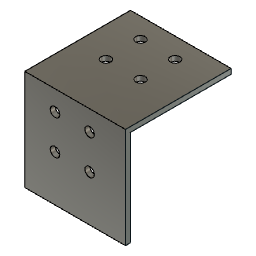
L brackets for Motors v5 (Autodesk Fusion 360 design; units mm, degrees)
Autodesk Fusion 360 part; units mm, degrees
sketch "Sketch1" plane through (0, 0, 0) normal (1, 0, 0) x (0, 1, 0)
  line L0 (0, 0) -> (2.54, 0)
  line L1 (2.54, 0) -> (2.54, 50.8)
  line L2 (2.54, 50.8) -> (0, 50.8)
  line L3 (0, 50.8) -> (0, 0)
  line L4 (0, 50.8) -> (53.34, 50.8)
  line L5 (53.34, 50.8) -> (53.34, 48.26)
  line L6 (53.34, 48.26) -> (0, 48.26)
  line L7 (0, 48.26) -> (0, 50.8)
  dimension "d5" = 2.54
  dimension "d6" = 50.8
  dimension "d7" = 53.34
  dimension "d8" = 2.54
  constraint horizontal L0
  constraint vertical L1
  constraint horizontal L2
  constraint vertical L3
  constraint coincident L0.start L3.end
  constraint horizontal L4
  constraint vertical L5
  constraint horizontal L6
  constraint vertical L7
  measures "d5" distance of L0.start L0.end
  measures "d6" distance of L0.start L2.end
  measures "d7" distance of L2.end L4.end
  measures "d8" distance of L2.end L6.end
extrude "Extrude1" add sketch "Sketch1" along normal blind 50.8 contours L1 L4 L5 L6
extrude "Extrude2" add sketch "Sketch1" along normal blind 50.8 contours L1 L2 L3 L4 L6 L7
extrude "Extrude3" add sketch "Sketch1" along normal blind 50.8 contours L0 L1 L3 L6
sketch "Sketch3" plane through (0, 0, 50.8) normal (0, 0, 1) x (-1, 0, 0)
  line L0 (0, -53.34) -> (0, 0)
  line L1 (0, 0) -> (-50.8, 0)
  line L2 (-50.8, 0) -> (-50.8, -53.34)
  line L3 (-50.8, -53.34) -> (0, -53.34)
  circle A0 centre (-15.24, -43.18) radius 2.3813
  circle A1 centre (-32.7025, -43.18) radius 2.3813
  circle A2 centre (-15.24, -25.7175) radius 2.3813
  circle A3 centre (-32.7025, -25.7175) radius 2.3813
  dimension "d15" = 17.4625
  dimension "d16" = 17.4625
  dimension "d17" = 4.7625
  dimension "d18" = 4.7625
  dimension "d19" = 4.7625
  dimension "d20" = 4.7625
  measures "d15" distance of A0.centre A1.centre
  measures "d16" distance of A0.centre A2.centre
  measures "d17" diameter of A0
  measures "d18" diameter of A1
  measures "d19" diameter of A2
  measures "d20" diameter of A3
hole "Hole1" at (32.7025, 43.18, 50.8) direction (0, 0, -1) diameter 4.7625 depth 22.86 tip angle 118
hole "Hole2" at (15.24, 43.18, 50.8) at (15.24, 25.7175, 50.8) at (32.7025, 25.7175, 50.8) direction (0, 0, -1) diameter 4.7752 depth 22.86 tip angle 118
sketch "Sketch4" plane through (0, 0, 0) normal (0, -1, 0) x (1, 0, 0)
  line L0 (0, 50.8) -> (0, 0)
  line L1 (0, 0) -> (50.8, 0)
  line L2 (50.8, 0) -> (50.8, 50.8)
  line L3 (50.8, 50.8) -> (0, 50.8)
  line L4 (0, 50.8) -> (15.2337, 50.8)
  line L5 (15.2337, 50.8) -> (15.2337, 40.6463)
  line L6 (15.2337, 40.6463) -> (32.6962, 40.6463)
  line L7 (32.6962, 40.6463) -> (32.6962, 23.1838)
  line L8 (32.6962, 23.1838) -> (15.2337, 23.1838)
  line L9 (15.2337, 23.1838) -> (15.2337, 40.6463)
  circle A0 centre (15.2337, 40.6463) radius 2.3812
  circle A1 centre (32.6962, 40.6463) radius 2.3812
  circle A2 centre (15.2337, 23.1838) radius 2.3813
  circle A3 centre (32.6962, 23.1838) radius 2.3812
  dimension "d42" = 15.2336
  dimension "d43" = 10.1537
  dimension "d44" = 17.4625
  dimension "d45" = 17.4625
  dimension "d46" = 4.7625
  dimension "d47" = 4.7625
  dimension "d48" = 4.7625
  dimension "d49" = 4.7625
  constraint coincident L0.start L3.end
  constraint perpendicular L0 L4
  constraint perpendicular L4 L5
  constraint horizontal L6
  constraint vertical L7
  constraint horizontal L8
  constraint vertical L9
  constraint coincident L5.end L6.start
  constraint coincident L6.end L7.start
  constraint coincident L8.end L9.start
  constraint coincident L7.end L8.start
  measures "d42" distance of L0.start L4.end
  measures "d43" distance of L4.end L5.end
  measures "d44" distance of L5.end L6.end
  measures "d45" distance of L5.end L8.end
  measures "d46" diameter of A0
  measures "d47" diameter of A1
  measures "d48" diameter of A2
  measures "d49" diameter of A3
hole "Hole3" at (15.2337, 0, 40.6463) at (15.2337, 0, 23.1838) at (32.6962, 0, 40.6463) at (32.6962, 0, 23.1838) direction (0, 1, 0) diameter 4.7752 depth 22.86 tip angle 118
sketch "Sketch6" plane through (50.8, 0, 0) normal (1, 0, 0) x (0, 1, 0)
  line L0 (53.34, 48.26) -> (53.34, 50.8)
  line L1 (53.34, 50.8) -> (0, 50.8)
  line L2 (0, 50.8) -> (0, 0)
  line L3 (0, 0) -> (2.54, 0)
  line L4 (2.54, 0) -> (2.54, 48.26)
  line L5 (2.54, 48.26) -> (53.34, 48.26)
equation "d15 = ( 11 / 16 ) * 1 in"
equation "d16 = ( 11 / 16 ) * 1 in"
equation "d17 = ( 3 / 16 ) * 1 in"
equation "d18 = ( 3 / 16 ) * 1 in"
equation "d19 = ( 3 / 16 ) * 1 in"
equation "d20 = ( 3 / 16 ) * 1 in"
equation "d42 = 0.506 in + ( 3 / 32 ) * 1 in"
equation "d43 = 0.306 in + ( 3 / 32 ) * 1 in"
equation "d44 = ( 11 / 16 ) * 1 in"
equation "d45 = ( 11 / 16 ) * 1 in"
equation "d46 = ( 3 / 16 ) * 1 in"
equation "d47 = ( 3 / 16 ) * 1 in"
equation "d48 = ( 3 / 16 ) * 1 in"
equation "d49 = ( 3 / 16 ) * 1 in"
